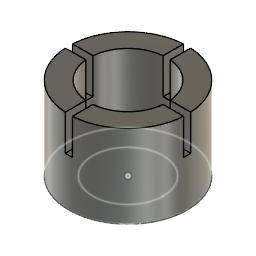
Final_rocket_mount_1 (Autodesk Fusion 360 design; units mm, degrees)
part number: 2026-05-01-17-17-46-245
Autodesk Fusion 360 part; units mm, degrees
sketch "Sketch1" plane through (0, 0, 0) normal (0, 0, 1) x (1, 0, 0)
  circle A0 centre (0, 0) radius 25
  circle A1 centre (0, 0) radius 14.8
  dimension "d1" = 50
  dimension "d8" = 29.6
  constraint coincident A0.centre A1.centre
  constraint concentric A0 A1
  measures "d1" diameter of A0
  measures "d8" diameter of A1
extrude "Extrude1" add sketch "Sketch1" along normal blind 10 contours A0 | A1
sketch "Sketch2" plane through (0, 0, 10) normal (0, 0, 1) x (-1, 0, 0)
  circle A0 centre (0, 0) radius 25
  circle A1 centre (0, 0) radius 16.375
  dimension "d5" = 32.75
  constraint coincident A0.centre A1.centre
  measures "d5" diameter of A1
extrude "Extrude2" cut sketch "Sketch2" against normal blind 6.75 contours A1
extrude "Extrude3" cut sketch "Sketch1" along normal blind 35 contours A1
extrude "Extrude4" add 1 faces at (21.971, -2.0555, 10) along direction (0, 0, 1) blind 10
sketch "Sketch3" plane through (0, 0, 20) normal (0, 0, 1) x (-1, 0, 0)
  circle A0 centre (0, 0) radius 16.375
  circle A1 centre (0, 0) radius 25
  circle A2 centre (0, 0) radius 25
  circle A3 centre (0, 0) radius 14.5357
  line L0 (-1.5, -16.3062) -> (-1.5, -24.955)
  line L1 (1.5, -16.3062) -> (1.5, -24.955)
  line L2 (16.3062, -1.5) -> (24.955, -1.5)
  line L3 (16.3062, 1.5) -> (24.955, 1.5)
  line L4 (1.5, 16.3062) -> (1.5, 24.955)
  line L5 (-1.5, 16.3062) -> (-1.5, 24.955)
  line L6 (-16.3062, 1.5) -> (-24.955, 1.5)
  line L7 (-16.3062, -1.5) -> (-24.955, -1.5)
  dimension "d16" = 360
  constraint coincident A0.centre A1.centre
  constraint concentric A2 A3
  constraint vertical L0
  constraint vertical L1
  constraint coincident A0 L1.start
  constraint coincident A0 L0.start
  constraint coincident A1 L0.end
  constraint coincident A1 L1.end
extrude "Extrude5" add sketch "Sketch3" along normal blind 15 contours A0 A1 A2 L3 L4 | A0 A1 A2 L1 L2 | A0 A1 A2 L5 L6 | A0 A1 A2 L0 L7
